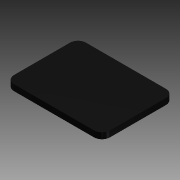
# Autodesk Inventor part: base
Saved by Autodesk Inventor 2015 (Build 190159000, 159)
## iProperties
Created: 2015-02-03
Part Number: base
Material: Generic
Document SubType Name: Modeling
Designer: rubidium
Density: 1 g/cm^3
Appearance: Default
Author: rubidium
Autodesk Inventor part; units mm, degrees
ref_plane "YZ Plane" through (0, 0, 0) normal (1, 0, 0) x (0, 1, 0)
ref_plane "XZ Plane" through (0, 0, 0) normal (0, 1, 0) x (-1, 0, 0)
ref_plane "XY Plane" through (0, 0, 0) normal (0, 0, 1) x (1, 0, 0)
sketch "Sketch1" plane through (0, 0, 0) normal (0, 1, 0) x (-1, 0, 0)
  line L0 (558.8, 0) -> (50.8, 0)
  line L1 (0, -50.8) -> (0, -406.4)
  line L2 (50.8, -457.2) -> (558.8, -457.2)
  line L3 (609.6, -406.4) -> (609.6, -50.8)
  arc A0 (609.6, -50.8) -> (558.8, 0) centre (558.8, -50.8) ccw
  arc A1 (558.8, -457.2) -> (609.6, -406.4) centre (558.8, -406.4) ccw
  arc A2 (0, -406.4) -> (50.8, -457.2) centre (50.8, -406.4) ccw
  arc A3 (50.8, 0) -> (0, -50.8) centre (50.8, -50.8) ccw
  point P0 (0, 0)
  point P1 (609.6, 0)
  point P2 (0, -457.2)
  point P3 (0, 0)
  point P4 (609.6, -457.2)
  dimension "d0" = 457.2
  dimension "d1" = 609.6
  dimension "d2" = 50.8
  constraints: 8 end point, 8 point on circle, 8 point on line, 8 tangent, 4 centre point, 3 equal radius, 2 parallel, 1 coincident, 1 horizontal, 1 perpendicular
  measures "d0" distance of point (609.6, -457.2) point (609.6, 0)
  measures "d1" distance of point (0, -457.2) point (609.6, -457.2)
  measures "d2" radius of A0
extrude "Extrusion1" add sketch "Sketch1" along normal blind 38.1
body "Solid1"
